Autodesk Fusion 360 part; units mm, degrees
(part 2 of 2)
fillet "Abrundung8" radius 2 20 edges at (32.15, 102, 2) (33.65, 181.85, 2) (35.15, 102, 2) (33.65, 22.15, 2) (99.3211, 187.7169, 2) (92.9417, 169.4744, 2) (87.3146, 150.6229, 2) (102, 150, 2) (116.6854, 150.6229, 2) (111.0583, 169.4743, 2) (104.679, 187.7168, 2) (102, 188, 2) (175.35, 181.85, 2) (173.85, 159.35, 2) (175.35, 136.85, 2) (176.85, 159.35, 2) (153.85, 44.65, 2) (155.35, 67.15, 2) (156.85, 44.65, 2) (155.35, 22.15, 2)
fillet "Abrundung9" radius 1 20 edges at (33.65, 181.85, 8.25) (32.15, 102, 8.25) (33.65, 22.15, 8.25) (35.15, 102, 8.25) (153.85, 44.65, 8.25) (155.35, 67.15, 8.25) (156.85, 44.65, 8.25) (155.35, 22.15, 8.25) (173.85, 159.35, 8.25) (175.35, 181.85, 8.25) (176.85, 159.35, 8.25) (175.35, 136.85, 8.25) (116.6854, 150.6229, 8.25) (111.0583, 169.4743, 8.25) (104.679, 187.7168, 8.25) (102, 188, 8.25) (99.3211, 187.7169, 8.25) (92.9417, 169.4744, 8.25) (87.3146, 150.6229, 8.25) (102, 150, 8.25)
chamfer "Fase2" distance 0.5 angle 45 2 edges at (78.1654, 83.452, 10) (121.7034, 121.773, 10)
